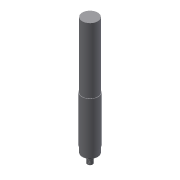
# Autodesk Inventor part: holdingRod
Saved by Autodesk Inventor 2015 (Build 190159000, 159)
## iProperties
Created: 2015-10-29
Part Number: holdingRod
Material: Generic
Document SubType Name: Modeling
Designer: jad211
Density: 1 g/cm^3
Appearance: Default
Author: jad211
Autodesk Inventor part; units mm, degrees
ref_plane "YZ Plane" through (0, 0, 0) normal (1, 0, 0) x (0, 1, 0)
ref_plane "XZ Plane" through (0, 0, 0) normal (0, 1, 0) x (-1, 0, 0)
ref_plane "XY Plane" through (0, 0, 0) normal (0, 0, 1) x (1, 0, 0)
sketch "Sketch1" plane through (0, 0, 0) normal (0, 1, 0) x (-1, 0, 0)
  line L0 (0, 0) -> (-5.9, 0)
  line L1 (-5.9, 0) -> (-5.9, -50)
  line L2 (-5.9, -50) -> (-6.3, -50)
  line L3 (-6.3, -50) -> (-6.3, -85)
  line L4 (-6.3, -85) -> (-5.9, -85)
  line L5 (-5.9, -85) -> (-5.9, -90)
  line L6 (-5.9, -90) -> (-2, -90)
  line L7 (-2, -90) -> (-2, -97)
  line L8 (-2, -97) -> (0, -97)
  line L9 (0, -97) -> (0, 0)
  dimension "d1" = 5.9
  dimension "d2" = 50
  dimension "d3" = 7
  dimension "d4" = 5
  dimension "d5" = 35
  dimension "d7" = 6.3
  dimension "d8" = 2
  constraints: 20 end point, 7 perpendicular, 2 point on line, 1 horizontal, 1 parallel
  measures "d1" distance of L0.start L0.end
  measures "d2" distance of L0.end L1.end
  measures "d3" distance of L6.end L7.end
  measures "d4" distance of L4.end L5.end
  measures "d5" distance of L2.end L3.end
  measures "d7" distance between parallel lines of L9 L3
  measures "d8" distance of L7.end L8.end
revolve "Revolution1" add sketch "Sketch1" angle 360 about axis through (0, 0, -97) along (0, 0, 1)
thread "Thread1" size "M4x0.7" class "6g" standard "ANSI Metric M Profile" full length
body "Solid1"
